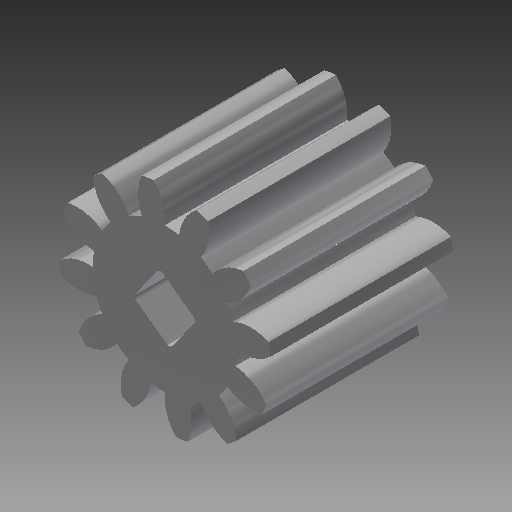
# Autodesk Inventor part: 276-2251
Saved by Autodesk Inventor 2017 (Build 210142000, 142)
## iProperties
Category: Motion
Company: Autodesk Inc.
Created: 2012-02-19
Part Number: 276-2251
Document SubType Name: Modeling
Designer: Autodesk Inc.
Density: 7.85 g/cm^3
Catalog Web Link: http://www.vexrobotics.com/276-2251.html
Description: 12 tooth spur gear
Vendor: VEX
Material: Steel
Mass: 11.4509 g
Surface Area: 14.3872 cm^2
Volume: 1.45871 cm^3
Appearance: Steel
d4: 0.000 in
d5: 0.000 in
Author: Autodesk Inc.
Autodesk Inventor part; units mm, degrees
ref_plane "YZ Plane" through (0, 0, 0) normal (1, 0, 0) x (0, 1, 0)
ref_plane "XZ Plane" through (0, 0, 0) normal (0, 1, 0) x (-1, 0, 0)
ref_plane "XY Plane" through (0, 0, 0) normal (0, 0, 1) x (1, 0, 0)
sketch "Sketch1" plane through (0, 0, 0) normal (0, 0, 1) x (1, 0, 0)
  arc A0 (0.7817, -7.3626) -> (1.5994, -7.2292) centre (0, 0) ccw
  arc A1 (1.5994, -7.2292) -> (1.5994, -4.7642) centre (-1.1357, -5.9967) ccw
  arc A2 (1.5994, -4.7642) -> (2.5111, -4.3532) centre (0, 0) ccw
  arc A3 (2.5111, -4.3532) -> (4.3583, -5.9854) centre (5.2457, -3.1197) ccw
  arc A4 (4.3583, -5.9854) -> (4.9997, -5.4609) centre (0, 0) ccw
  arc A5 (4.9997, -5.4609) -> (3.7672, -3.3262) centre (2.0148, -5.7611) ccw
  arc A6 (3.7672, -3.3262) -> (4.3512, -2.5144) centre (0, 0) ccw
  arc A7 (4.3512, -2.5144) -> (6.7671, -3.0044) centre (6.1028, -0.0788) ccw
  arc A8 (6.7671, -3.0044) -> (7.0604, -2.2294) centre (0, 0) ccw
  arc A9 (7.0604, -2.2294) -> (4.9256, -0.9969) centre (4.6254, -3.9819) ccw
  arc A10 (4.9256, -0.9969) -> (5.0255, -0.0019) centre (0, 0) ccw
  arc A11 (5.0255, -0.0019) -> (7.3626, 0.7817) centre (5.3246, 2.9831) ccw
  arc A12 (7.3626, 0.7817) -> (7.2292, 1.5994) centre (0, 0) ccw
  arc A13 (7.2292, 1.5994) -> (4.7642, 1.5994) centre (5.9967, -1.1357) ccw
  arc A14 (4.7642, 1.5994) -> (4.3532, 2.5111) centre (0, 0) ccw
  arc A15 (4.3532, 2.5111) -> (5.9854, 4.3583) centre (3.1197, 5.2457) ccw
  arc A16 (5.9854, 4.3583) -> (5.4609, 4.9997) centre (0, 0) ccw
  arc A17 (5.4609, 4.9997) -> (3.3262, 3.7672) centre (5.7611, 2.0148) ccw
  arc A18 (3.3262, 3.7672) -> (2.5144, 4.3512) centre (0, 0) ccw
  arc A19 (2.5144, 4.3512) -> (3.0044, 6.7671) centre (0.0788, 6.1028) ccw
  arc A20 (3.0044, 6.7671) -> (2.2294, 7.0604) centre (0, 0) ccw
  arc A21 (2.2294, 7.0604) -> (0.9969, 4.9256) centre (3.9819, 4.6254) ccw
  arc A22 (0.9969, 4.9256) -> (0.0019, 5.0255) centre (0, 0) ccw
  arc A23 (0.0019, 5.0255) -> (-0.7817, 7.3626) centre (-2.9831, 5.3246) ccw
  arc A24 (-0.7817, 7.3626) -> (-1.5994, 7.2292) centre (0, 0) ccw
  arc A25 (-1.5994, 7.2292) -> (-1.5994, 4.7642) centre (1.1357, 5.9967) ccw
  arc A26 (-1.5994, 4.7642) -> (-2.5111, 4.3532) centre (0, 0) ccw
  arc A27 (-2.5111, 4.3532) -> (-4.3583, 5.9854) centre (-5.2457, 3.1197) ccw
  arc A28 (-4.3583, 5.9854) -> (-4.9997, 5.4609) centre (0, 0) ccw
  arc A29 (-4.9997, 5.4609) -> (-3.7672, 3.3262) centre (-2.0148, 5.7611) ccw
  arc A30 (-3.7672, 3.3262) -> (-4.3512, 2.5144) centre (0, 0) ccw
  arc A31 (-4.3512, 2.5144) -> (-6.7671, 3.0044) centre (-6.1028, 0.0788) ccw
  arc A32 (-6.7671, 3.0044) -> (-7.0604, 2.2294) centre (0, 0) ccw
  arc A33 (-7.0604, 2.2294) -> (-4.9256, 0.9969) centre (-4.6254, 3.9819) ccw
  arc A34 (-4.9256, 0.9969) -> (-5.0255, 0.0019) centre (0, 0) ccw
  arc A35 (-5.0255, 0.0019) -> (-7.3626, -0.7817) centre (-5.3246, -2.9831) ccw
  arc A36 (-7.3626, -0.7817) -> (-7.2292, -1.5994) centre (0, 0) ccw
  arc A37 (-7.2292, -1.5994) -> (-4.7642, -1.5994) centre (-5.9967, 1.1357) ccw
  arc A38 (-4.7642, -1.5994) -> (-4.3532, -2.5111) centre (0, 0) ccw
  arc A39 (-4.3532, -2.5111) -> (-5.9854, -4.3583) centre (-3.1197, -5.2457) ccw
  arc A40 (-5.9854, -4.3583) -> (-5.4609, -4.9997) centre (0, 0) ccw
  arc A41 (-5.4609, -4.9997) -> (-3.3262, -3.7672) centre (-5.7611, -2.0148) ccw
  arc A42 (-3.3262, -3.7672) -> (-2.5144, -4.3512) centre (0, 0) ccw
  arc A43 (-2.5144, -4.3512) -> (-3.0044, -6.7671) centre (-0.0788, -6.1028) ccw
  arc A44 (-3.0044, -6.7671) -> (-2.2294, -7.0604) centre (0, 0) ccw
  arc A45 (-2.2294, -7.0604) -> (-0.9969, -4.9256) centre (-3.9819, -4.6254) ccw
  arc A46 (-0.9969, -4.9256) -> (-0.0019, -5.0255) centre (0, 0) ccw
  arc A47 (-0.0019, -5.0255) -> (0.7817, -7.3626) centre (2.9831, -5.3246) ccw
  arc A48 (0.1554, -2.0674) -> (0.5099, -2.0096) centre (0.3037, -1.8612) ccw
  line L0 (0.1554, -2.0674) -> (-2.0096, -0.5099)
  arc A49 (-2.0674, -0.1554) -> (-2.0096, -0.5099) centre (-1.8612, -0.3037) ccw
  line L1 (-2.0674, -0.1554) -> (-0.5099, 2.0096)
  arc A50 (-0.1554, 2.0674) -> (-0.5099, 2.0096) centre (-0.3037, 1.8612) ccw
  line L2 (-0.1554, 2.0674) -> (2.0096, 0.5099)
  arc A51 (2.0674, 0.1554) -> (2.0096, 0.5099) centre (1.8612, 0.3037) ccw
  line L3 (2.0674, 0.1554) -> (0.5099, -2.0096)
  constraints: 104 point on circle, 52 centre point, 8 end point
extrude "Extrusion1" add sketch "Sketch1" against normal blind 12.7
sketch "Sketch2" plane through (0, 0, 0) normal (0, 0, 1) x (1, 0, 0)
  arc A0 (-0.9969, -4.9256) -> (-0.0019, -5.0255) centre (0, 0) ccw projected
  circle A1 centre (0, 0) radius 1.5875
  constraints: 1 centre point, 1 coincident
surface extrude "ExtrusionSrf1" sketch "Sketch2" against normal up to surface (12.7 mm away) shown no curves A1
body "Solid1"
body "Srf1"
